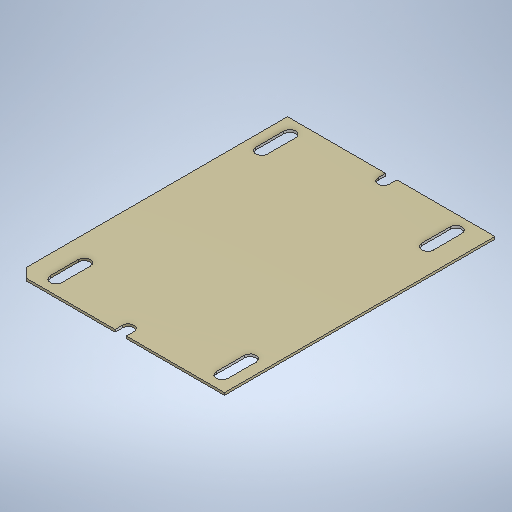
# Autodesk Inventor part: etl standard baseplate with cutouts
Saved by Autodesk Inventor 2025 (Build 290162000, 162)
## iProperties
Created: 2021-07-27
Part Number: etl standard baseplate with cutouts
Material: Generic
Document SubType Name: Modeling
Designer: Caleb
Density: 1 g/cm^3
Appearance: Default
Sending System: Autodesk Inventor 2022
Preprocessor: ST-DEVELOPER v18.1
Title: C:\Users\Caleb\Desktop\etl standard baseplate.stp
Author: Caleb
Autodesk Inventor part; units mm, degrees
ref_plane "YZ Plane" through (0, 0, 0) normal (1, 0, 0) x (0, 1, 0)
ref_plane "XZ Plane" through (0, 0, 0) normal (0, 1, 0) x (-1, 0, 0)
ref_plane "XY Plane" through (0, 0, 0) normal (0, 0, 1) x (1, 0, 0)
sketch "Sketch2" plane through (0, 0, 0) normal (0, 1, 0) x (-1, 0, 0)
  line L0 (-22.05, -28.75) -> (22.05, -28.75)
  line L1 (22.05, -28.75) -> (22.05, 28.75)
  line L2 (22.05, 28.75) -> (-22.05, 28.75)
  line L3 (-22.05, 28.75) -> (-22.05, -28.75)
  line L4 (-22.05, -28.75) -> (22.05, 28.75) construction
  line L5 (22.05, -28.75) -> (-22.05, 28.75) construction
  point P0 (0, 0)
  dimension "d28" = 44.1
  dimension "d29" = 57.5
  constraints: 12 end point, 2 midpoint, 2 parallel, 1 horizontal, 1 perpendicular
  measures "d28" distance of L1.end L2.end
  measures "d29" distance of L0.end L1.end
extrude "Extrusion2" add sketch "Sketch2" along normal blind 0.5
sketch "Sketch3" plane through (0, 0.5, 0) normal (0, 1, 0) x (1, 0, 0)
  line L0 (3.17, 0) -> (-3.4256, 0) construction
  line L1 (-18, -28.75) -> (-18, -19.75)
  line L2 (-15.5, -19.75) -> (-15.5, -28.75)
  arc A0 (-15.5, -19.75) -> (-18, -19.75) centre (-16.75, -19.75) ccw
  line L3 (-22.05, -28.75) -> (22.05, -28.75) projected
  line L4 (-22.05, 28.75) -> (-22.05, -28.75) projected
  line L5 (19.8, -28.75) -> (19.8, -19.75)
  line L6 (17.3, -19.75) -> (17.3, -28.75)
  arc A1 (19.8, -19.75) -> (17.3, -19.75) centre (18.55, -19.75) ccw
  line L7 (15.5, 28.75) -> (15.5, 19.75)
  line L8 (22.05, 28.75) -> (-22.05, 28.75) projected
  line L9 (18, 28.75) -> (18, 19.75)
  arc A2 (15.5, 19.75) -> (18, 19.75) centre (16.75, 19.75) ccw
  line L10 (22.05, -28.75) -> (22.05, 28.75) projected
  line L11 (-19.8, 28.75) -> (-19.8, 19.75)
  line L12 (-17.3, 28.75) -> (-17.3, 19.75)
  arc A3 (-19.8, 19.75) -> (-17.3, 19.75) centre (-18.55, 19.75) ccw
  point P0 (0, 0)
  point P1 (10.634, -28.75)
  point P2 (12.3949, -28.75)
  dimension "d32" = 2.5
  dimension "d33" = 9
  dimension "d34" = 1.25
  dimension "d48" = 5.3
  dimension "d60" = 9
  dimension "d61" = 9
  dimension "d62" = 1.25
  dimension "d64" = 9
  dimension "d65" = 9
  dimension "d66" = 1.25
  dimension "d71" = 3.5
  dimension "d87" = 5.3
  dimension "d88" = 3.5
  constraints: 18 end point, 8 point on circle, 7 point on line, 5 parallel, 4 centre point, 4 vertical, 3 horizontal alignment, 2 perpendicular, 1 equal radius, 1 horizontal, 1 tangent
  measures "d32" distance between parallel lines of L1 L2
  measures "d33" distance of L1.start L1.end
  measures "d34" radius of A0
  measures "d48" distance from line of L4 A0.centre
  measures "d60" distance of L7.start L7.end
  measures "d61" distance of L9.start L9.end
  measures "d62" radius of A2
  measures "d64" distance of L11.start L11.end
  measures "d65" distance of L12.start L12.end
  measures "d66" radius of A3
  measures "d71" distance from line of L4 A3.centre
  measures "d87" distance from line of L10 A2.centre
  measures "d88" distance from line of L10 A1.centre
extrude "Extrusion3" cut sketch "Sketch3" against normal through all contours L1 A0 L2 L3 | L6 A1 L5 L3 | L8 L12 A3 L11 | L8 L9 A2 L7
sketch "Sketch4" plane through (0, 0.5, 0) normal (0, 1, 0) x (1, 0, 0)
  line L0 (-22.05, 28.75) -> (-22.05, -28.75) projected
  line L1 (-22.05, -28.75) -> (22.05, -28.75) projected
  line L2 (22.05, -28.75) -> (22.05, 28.75) projected
  line L3 (22.05, 28.75) -> (-22.05, 28.75) projected
  point P0 (0, 0)
  point P1 (0, -27.15)
  point P2 (0, 27.15)
  point P3 (-18, -28.75)
  point P4 (-12.775, 28.75)
  dimension "d37" = 22.05
  dimension "d38" = 1.6
  dimension "d40" = 1.6
  dimension "d68" = 44.1
  constraints: 1 vertical alignment
  measures "d37" distance from line of L0 point (0, -27.15)
  measures "d38" distance from line of L1 point (0, -27.15)
  measures "d40" distance from line of L3 point (0, 27.15)
  measures "d68" distance of L0.end L1.end
hole "Hole1" at (0, 0.5, 27.15) at (0, 0.5, -27.15) direction (0, -1, 0) diameter 2.4 end through all clearance for "Flat Head Machine Screw" size "M2" standard "Ansi Metric M Profile"
sketch "Sketch5" plane through (0, 0.5, 0) normal (0, 1, 0) x (1, 0, 0)
  line L0 (-22.05, -28.75) -> (-18, -28.75) projected
  line L1 (-20.05, -28.75) -> (-22.05, -26.75)
  line L2 (-22.05, 28.75) -> (-22.05, -28.75) projected
  point P0 (0, 0)
  dimension "d49" = 2
  dimension "d50" = 2
  constraints: 2 end point, 2 point on line
  measures "d49" distance of L0.start L1.start
  measures "d50" distance of L0.start L1.end
extrude "Extrusion4" cut sketch "Sketch5" against normal through all
sketch "Sketch6" plane through (0, 0.5, 0) normal (0, 1, 0) x (1, 0, 0)
  circle A0 centre (0, -27.15) radius 1.2 projected
  line L0 (-1.2, -27.15) -> (-1.2, -28.75)
  line L1 (-15.5, -28.75) -> (17.3, -28.75) projected
  line L2 (1.2, -27.15) -> (1.2, -28.75)
  line L3 (1.2, -27.15) -> (-1.2, -27.15)
  line L4 (24.0299, 0) -> (-42.1887, 0)
  line L5 (-1.2, 27.15) -> (-1.2, 28.75)
  line L6 (1.2, 27.15) -> (1.2, 28.75)
  line L7 (1.2, 27.15) -> (-1.2, 27.15)
  line L8 (15.5, 28.75) -> (-17.3, 28.75) projected
  point P0 (0, 0)
  point P1 (0, 27.15)
  constraints: 14 end point, 5 symmetric about line, 2 horizontal, 2 horizontal alignment, 2 point on circle, 2 point on line, 2 vertical
extrude "Extrusion5" cut sketch "Sketch6" against normal through all contours L2 L1 L0 A0 | L5 L8 L6 L7
sketch "Sketch7" plane through (0, 0.5, 0) normal (0, 1, 0) x (1, 0, 0)
  line L0 (-15.5, -19.75) -> (-15.5, -28.75) projected
  arc A0 (-18, -25.75) -> (-15.5, -25.75) centre (-16.75, -25.75) ccw
  line L1 (-18, -28.75) -> (-18, -19.75) projected
  arc A1 (-15.5, -19.75) -> (-18, -19.75) centre (-16.75, -19.75) ccw projected
  line L2 (-15.5, -28.75) -> (-1.2, -28.75) projected
  line L3 (-18, -28.75) -> (-15.5, -28.75)
  arc A2 (17.3, -25.75) -> (19.8, -25.75) centre (18.55, -25.75) ccw
  line L4 (17.3, -28.75) -> (17.3, -19.75) projected
  line L5 (19.8, -19.75) -> (19.8, -28.75) projected
  line L6 (1.2, -28.75) -> (17.3, -28.75) projected
  line L7 (17.3, -28.75) -> (19.8, -28.75)
  line L8 (-17.3, 28.75) -> (-17.3, 19.75) projected
  line L9 (-19.8, 19.75) -> (-19.8, 28.75) projected
  arc A3 (-17.3, 25.75) -> (-19.8, 25.75) centre (-18.55, 25.75) ccw
  line L10 (-1.2, 28.75) -> (-17.3, 28.75) projected
  line L11 (15.5, 28.75) -> (1.2, 28.75) projected
  arc A4 (18, 25.75) -> (15.5, 25.75) centre (16.75, 25.75) ccw
  line L12 (15.5, 19.75) -> (15.5, 28.75) projected
  line L13 (18, 28.75) -> (18, 19.75) projected
  line L14 (-19.8, 28.75) -> (-17.3, 28.75)
  line L15 (15.5, 28.75) -> (18, 28.75)
  point P0 (0, 0)
  dimension "d73" = 1.25
  dimension "d74" = 1.25
  dimension "d75" = 3
  dimension "d78" = 1.25
  dimension "d80" = 3
  dimension "d81" = 1.25
  dimension "d82" = 3
  dimension "d85" = 1.25
  dimension "d86" = 3
  constraints: 8 end point, 8 point on circle, 8 point on line, 4 centre point, 3 horizontal, 2 horizontal alignment, 1 collinear
  measures "d73" radius of A0
  measures "d74" radius of A1
  measures "d75" vertical distance of L1.start A0.centre
  measures "d78" radius of A2
  measures "d80" distance from line of L6 A2.centre
  measures "d81" radius of A3
  measures "d82" distance from line of L10 A3.centre
  measures "d85" radius of A4
  measures "d86" distance from line of L11 A4.centre
extrude "Extrusion6" add sketch "Sketch7" against normal up to surface (0.5 mm away) contours L0 L3 L1 A0 | A2 L5 L7 L4 | L8 A3 L9 L14 | A4 L12 L15 L13
equation "\"d34\" = 0.5 * d32"
equation "\"d60\" = d33"
equation "\"d61\" = d33"
equation "\"d62\" = d34"
equation "\"d64\" = d33"
equation "\"d65\" = d33"
equation "\"d66\" = d34"
equation "\"d87\" = d48"
equation "\"d88\" = d71"
equation "\"d37\" = 0.5 * d68"
equation "\"d40\" = d38"
equation "\"d73\" = d74"
equation "\"d78\" = d79"
equation "\"d80\" = d75"
equation "\"d81\" = d74"
equation "\"d82\" = d75"
equation "\"d85\" = d74"
equation "\"d86\" = d75"
equation "\"d79\" = 1.25"
body "Solid3"
